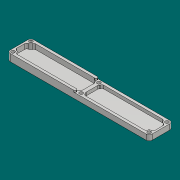
# Autodesk Inventor part: delay_spacer
Saved by Autodesk Inventor 2018.2 (Build 222227000, 227)
## iProperties
Created: 2021-05-04
Part Number: delay_spacer
Material: アルミニウム 6061
Document SubType Name: Modeling
Designer: gisen
Density: 2.7 g/cm^3
Appearance: アルミニウム - フラット
Author: gisen
Autodesk Inventor part; units mm, degrees
ref_plane "YZ Plane" through (0, 0, 0) normal (1, 0, 0) x (0, 1, 0)
ref_plane "XZ Plane" through (0, 0, 0) normal (0, 1, 0) x (-1, 0, 0)
ref_plane "XY Plane" through (0, 0, 0) normal (0, 0, 1) x (1, 0, 0)
sketch "スケッチ1" plane through (0, 0, 0) normal (0, 0, 1) x (1, 0, 0)
  line L0 (0, 0) -> (125.3, 0) construction
  line L1 (125.3, 0) -> (125.3, 16.35) construction
  line L2 (125.3, 16.35) -> (0, 16.35) construction
  line L3 (0, 16.35) -> (0, 0) construction
  line L4 (62.65, 16.35) -> (62.65, 0) construction
  line L5 (-2.7, 19.05) -> (128, 19.05) construction
  line L6 (128, 19.05) -> (128, -2.7) construction
  line L7 (128, -2.7) -> (-2.7, -2.7) construction
  line L8 (-2.7, -2.7) -> (-2.7, 19.05) construction
  circle A0 centre (0, 16.35) radius 1.6
  circle A1 centre (0, 0) radius 1.6
  circle A2 centre (62.65, 16.35) radius 1.6
  circle A3 centre (62.65, 0) radius 1.6
  circle A4 centre (125.3, 0) radius 1.6
  circle A5 centre (125.3, 16.35) radius 1.6
  arc A6 (0, 19.05) -> (-2.7, 16.35) centre (0, 16.35) ccw
  arc A7 (-2.7, 0) -> (0, -2.7) centre (0, 0) ccw
  arc A8 (128, 16.35) -> (125.3, 19.05) centre (125.3, 16.35) ccw
  arc A9 (125.3, -2.7) -> (128, 0) centre (125.3, 0) ccw
  line L9 (0, 19.05) -> (125.3, 19.05)
  line L10 (-2.7, 16.35) -> (-2.7, 0)
  line L11 (0, -2.7) -> (125.3, -2.7)
  line L12 (128, 0) -> (128, 16.35)
  arc A10 (0, 13.65) -> (2.7, 16.35) centre (0, 16.35) ccw
  line L13 (0, 13.65) -> (-1.1, 13.65)
  line L14 (-1.1, 13.65) -> (-1.1, 2.7)
  line L15 (-1.1, 2.7) -> (0, 2.7)
  arc A11 (2.7, 0) -> (0, 2.7) centre (0, 0) ccw
  line L16 (2.7, 16.35) -> (2.7, 16.65)
  line L17 (2.7, 16.65) -> (59.95, 16.65)
  line L18 (59.95, 16.65) -> (59.95, 16.35)
  arc A12 (59.95, 16.35) -> (61.05, 14.1751) centre (62.65, 16.35) ccw
  line L19 (61.05, 14.1751) -> (61.05, 2.1749)
  arc A13 (61.05, 2.1749) -> (59.95, 0) centre (62.65, 0) ccw
  line L20 (2.7, 0) -> (2.7, -0.3)
  line L21 (2.7, -0.3) -> (59.95, -0.3)
  line L22 (59.95, -0.3) -> (59.95, 0)
  arc A14 (122.6, 16.35) -> (125.3, 13.65) centre (125.3, 16.35) ccw
  line L23 (125.3, 13.65) -> (126.4, 13.65)
  line L24 (126.4, 13.65) -> (126.4, 2.7)
  line L25 (126.4, 2.7) -> (125.3, 2.7)
  arc A15 (125.3, 2.7) -> (122.6, 0) centre (125.3, 0) ccw
  line L26 (122.6, 16.35) -> (122.6, 16.65)
  line L27 (122.6, 16.65) -> (65.35, 16.65)
  line L28 (65.35, 16.65) -> (65.35, 16.35)
  arc A16 (64.25, 14.1751) -> (65.35, 16.35) centre (62.65, 16.35) ccw
  line L29 (64.25, 14.1751) -> (64.25, 2.1749)
  arc A17 (65.35, 0) -> (64.25, 2.1749) centre (62.65, 0) ccw
  line L30 (122.6, 0) -> (122.6, -0.3)
  line L31 (122.6, -0.3) -> (65.35, -0.3)
  line L32 (65.35, -0.3) -> (65.35, 0)
  dimension "d0" = 125.3
  dimension "d1" = 16.35
  dimension "d2" = 2.7
  dimension "d3" = 3.2
  dimension "d4" = 1.6
  dimension "d5" = 1.6
  dimension "d6" = 2.4
  dimension "d7" = 2.4
  constraints: 66 end point, 24 point on circle, 18 centre point, 16 symmetric about line, 15 point on line, 14 coincident, 10 perpendicular, 9 equal radius, 4 parallel, 4 tangent, 3 vertical, 2 collinear, 2 horizontal, 2 midpoint, 7 other
  measures "d0" distance of L1.end L2.end
  measures "d1" distance of L0.end L1.end
  measures "d2" distance between parallel lines of L2 L5
  measures "d3" diameter of A0
  measures "d4" distance between parallel lines of L4 L19
  measures "d5" distance between parallel lines of L8 L14
  measures "d6" distance between parallel lines of L5 L17
  measures "d7" distance between parallel lines of L11 L21
extrude "押し出し1" add sketch "スケッチ1" along normal blind 5
sketch "スケッチ2" plane through (0, 0, 5) normal (0, 0, 1) x (1, 0, 0)
  arc A0 (122.6, 16.35) -> (125.3, 13.65) centre (125.3, 16.35) ccw projected
  line L0 (125.3, 13.65) -> (126.4, 13.65) projected
  line L1 (126.4, 13.65) -> (126.4, 2.7) projected
  line L2 (126.4, 2.7) -> (125.3, 2.7) projected
  arc A1 (125.3, 2.7) -> (122.6, 0) centre (125.3, 0) ccw projected
  line L3 (122.6, 0) -> (122.6, -0.3) projected
  line L4 (122.6, -0.3) -> (65.35, -0.3) projected
  line L5 (65.35, -0.3) -> (65.35, 0) projected
  arc A2 (65.35, 0) -> (64.25, 2.1749) centre (62.65, 0) ccw projected
  line L6 (64.25, 2.1749) -> (64.25, 14.1751) projected
  arc A3 (64.25, 14.1751) -> (65.35, 16.35) centre (62.65, 16.35) ccw projected
  line L7 (65.35, 16.35) -> (65.35, 16.65) projected
  line L8 (65.35, 16.65) -> (122.6, 16.65) projected
  line L9 (122.6, 16.65) -> (122.6, 16.35) projected
  line L10 (2.7, 16.35) -> (2.7, 16.65) projected
  line L11 (2.7, 16.65) -> (59.95, 16.65) projected
  line L12 (59.95, 16.65) -> (59.95, 16.35) projected
  arc A4 (59.95, 16.35) -> (61.05, 14.1751) centre (62.65, 16.35) ccw projected
  line L13 (61.05, 14.1751) -> (61.05, 2.1749) projected
  arc A5 (61.05, 2.1749) -> (59.95, 0) centre (62.65, 0) ccw projected
  line L14 (59.95, 0) -> (59.95, -0.3) projected
  line L15 (59.95, -0.3) -> (2.7, -0.3) projected
  line L16 (2.7, -0.3) -> (2.7, 0) projected
  arc A6 (2.7, 0) -> (0, 2.7) centre (0, 0) ccw projected
  line L17 (0, 2.7) -> (-1.1, 2.7) projected
  line L18 (-1.1, 2.7) -> (-1.1, 13.65) projected
  line L19 (-1.1, 13.65) -> (0, 13.65) projected
  arc A7 (0, 13.65) -> (2.7, 16.35) centre (0, 16.35) ccw projected
  circle A8 centre (125.3, 16.35) radius 1.6 projected
  circle A9 centre (125.3, 0) radius 1.6 projected
  circle A10 centre (62.65, 0) radius 1.6 projected
  circle A11 centre (62.65, 16.35) radius 1.6 projected
  circle A12 centre (0, 0) radius 1.6 projected
  circle A13 centre (0, 16.35) radius 1.6 projected
  arc A14 (0, 19.05) -> (-2.7, 16.35) centre (0, 16.35) ccw projected
  line L20 (-2.7, 16.35) -> (-2.7, 0) projected
  arc A15 (-2.7, 0) -> (0, -2.7) centre (0, 0) ccw projected
  line L21 (0, -2.7) -> (125.3, -2.7) projected
  arc A16 (125.3, -2.7) -> (128, 0) centre (125.3, 0) ccw projected
  line L22 (128, 0) -> (128, 16.35) projected
  arc A17 (128, 16.35) -> (125.3, 19.05) centre (125.3, 16.35) ccw projected
  line L23 (125.3, 19.05) -> (0, 19.05) projected
  line L24 (59.65, 19.05) -> (59.65, 16.65)
  line L25 (59.65, -0.3) -> (59.65, -2.7)
  dimension "d10" = 3
  dimension "d11" = 3
  constraints: 4 end point, 4 point on line, 1 collinear, 1 vertical
  measures "d10" distance from line of A3.centre L24
  measures "d11" distance from line of A2.centre L25
extrude "押し出し2" add sketch "スケッチ2" along normal blind 1.6 contours A7 L19 L18 L17 A6 L16 L15 L25 L21 A15 L20 A14 L23 L24 L11 L10
fillet "フィレット1" radius 2 16 edges at (122.6, -0.3, 2.5) (126.4, 2.7, 2.5) (126.4, 13.65, 2.5) (122.6, 16.65, 2.5) (65.35, 16.65, 2.5) (64.25, 14.1751, 2.5) (65.35, -0.3, 2.5) (64.25, 2.1749, 2.5) (61.05, 2.1749, 2.5) (59.95, -0.3, 2.5) (61.05, 14.1751, 2.5) (59.95, 16.65, 2.5) (2.7, 16.65, 3.3) (-1.1, 13.65, 3.3) (-1.1, 2.7, 3.3) (2.7, -0.3, 3.3)
fillet "フィレット2" radius 1 4 edges at (59.65, 19.05, 5.8) (59.65, 16.0959, 5.8) (59.65, 0.2541, 5.8) (59.65, -2.7, 5.8)
sketch "スケッチ3" plane through (0, 0, 0) normal (0, 0, -1) x (-1, 0, 0)
  arc A0 (-124.783, 13.7) -> (-122.7828, 15.3734) centre (-125.3, 16.35) ccw projected
  arc A1 (-120.9182, 16.65) -> (-122.7828, 15.3734) centre (-120.9182, 14.65) ccw projected
  line L0 (-120.9182, 16.65) -> (-67.0318, 16.65) projected
  arc A2 (-65.1672, 15.3734) -> (-67.0318, 16.65) centre (-67.0318, 14.65) ccw projected
  arc A3 (-65.1672, 15.3734) -> (-64.7181, 14.6142) centre (-62.65, 16.35) ccw projected
  arc A4 (-64.25, 13.3284) -> (-64.7181, 14.6142) centre (-66.25, 13.3284) ccw projected
  line L1 (-64.25, 13.3284) -> (-64.25, 3.0216) projected
  arc A5 (-64.7181, 1.7358) -> (-64.25, 3.0216) centre (-66.25, 3.0216) ccw projected
  arc A6 (-64.7181, 1.7358) -> (-65.1672, 0.9766) centre (-62.65, 0) ccw projected
  arc A7 (-67.0318, -0.3) -> (-65.1672, 0.9766) centre (-67.0318, 1.7) ccw projected
  line L2 (-67.0318, -0.3) -> (-120.9182, -0.3) projected
  arc A8 (-122.7828, 0.9766) -> (-120.9182, -0.3) centre (-120.9182, 1.7) ccw projected
  arc A9 (-122.7828, 0.9766) -> (-124.783, 2.65) centre (-125.3, 0) ccw projected
  arc A10 (-126.4, 4.613) -> (-124.783, 2.65) centre (-124.4, 4.613) ccw projected
  line L3 (-126.4, 4.613) -> (-126.4, 11.737) projected
  arc A11 (-124.783, 13.7) -> (-126.4, 11.737) centre (-124.4, 11.737) ccw projected
  arc A12 (-58.2682, 16.65) -> (-60.1328, 15.3734) centre (-58.2682, 14.65) ccw projected
  line L4 (-58.2682, 16.65) -> (-4.3818, 16.65) projected
  arc A13 (-2.5172, 15.3734) -> (-4.3818, 16.65) centre (-4.3818, 14.65) ccw projected
  arc A14 (-2.5172, 15.3734) -> (-0.517, 13.7) centre (0, 16.35) ccw projected
  arc A15 (1.1, 11.737) -> (-0.517, 13.7) centre (-0.9, 11.737) ccw projected
  line L5 (1.1, 11.737) -> (1.1, 4.613) projected
  arc A16 (-0.517, 2.65) -> (1.1, 4.613) centre (-0.9, 4.613) ccw projected
  arc A17 (-0.517, 2.65) -> (-2.5172, 0.9766) centre (0, 0) ccw projected
  arc A18 (-4.3818, -0.3) -> (-2.5172, 0.9766) centre (-4.3818, 1.7) ccw projected
  line L6 (-4.3818, -0.3) -> (-58.2682, -0.3) projected
  arc A19 (-60.1328, 0.9766) -> (-58.2682, -0.3) centre (-58.2682, 1.7) ccw projected
  arc A20 (-60.1328, 0.9766) -> (-60.5819, 1.7358) centre (-62.65, 0) ccw projected
  arc A21 (-61.05, 3.0216) -> (-60.5819, 1.7358) centre (-59.05, 3.0216) ccw projected
  line L7 (-61.05, 3.0216) -> (-61.05, 13.3284) projected
  arc A22 (-60.5819, 14.6142) -> (-61.05, 13.3284) centre (-59.05, 13.3284) ccw projected
  arc A23 (-60.5819, 14.6142) -> (-60.1328, 15.3734) centre (-62.65, 16.35) ccw projected
  circle A24 centre (-125.3, 16.35) radius 1.6 projected
  circle A25 centre (-125.3, 0) radius 1.6 projected
  circle A26 centre (-62.65, 0) radius 1.6 projected
  circle A27 centre (-62.65, 16.35) radius 1.6 projected
  circle A28 centre (0, 0) radius 1.6 projected
  circle A29 centre (0, 16.35) radius 1.6 projected
  arc A30 (2.7, 16.35) -> (0, 19.05) centre (0, 16.35) ccw projected
  line L8 (-125.3, 19.05) -> (0, 19.05) projected
  arc A31 (-125.3, 19.05) -> (-128, 16.35) centre (-125.3, 16.35) ccw projected
  line L9 (-128, 0) -> (-128, 16.35) projected
  arc A32 (-128, 0) -> (-125.3, -2.7) centre (-125.3, 0) ccw projected
  line L10 (0, -2.7) -> (-125.3, -2.7) projected
  arc A33 (0, -2.7) -> (2.7, 0) centre (0, 0) ccw projected
  line L11 (2.7, 16.35) -> (2.7, 0) projected
extrude "押し出し3" add sketch "スケッチ3" against normal blind 2 contours A0 A1 L0 A2 A3 A4 L1 A5 A6 A7 L2 A8 A9 A10 L3 A11 | L4 A13 A14 A15 L5 A16 A17 A18 L6 A19 A20 A21 L7 A22 A23 A12
equation "\"d7\" = d6"
equation "\"d11\" = d10"
